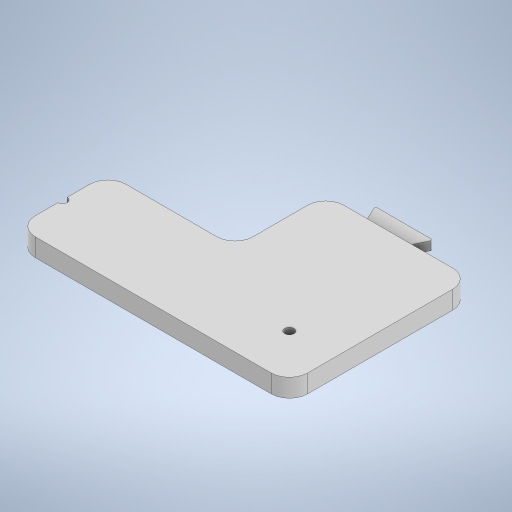
# Autodesk Inventor part: Area nh
Saved by Autodesk Inventor 2024 (Build 280153000, 153)
## iProperties
Created: 2024-03-01
Part Number: Area nh
Material: Generic
Document SubType Name: Modeling
Designer: laura
Density: 1 g/cm^3
Appearance: Default
Author: laura
Autodesk Inventor part; units mm, degrees
ref_plane "YZ Plane" through (0, 0, 0) normal (1, 0, 0) x (0, 1, 0)
ref_plane "XZ Plane" through (0, 0, 0) normal (0, 1, 0) x (-1, 0, 0)
ref_plane "XY Plane" through (0, 0, 0) normal (0, 0, 1) x (1, 0, 0)
sketch "Sketch1" plane through (0, 0, 0) normal (0, 1, 0) x (-1, 0, 0)
  line L0 (0, 0) -> (200, 0)
  line L1 (200, 0) -> (200, -150)
  line L2 (200, -150) -> (0, -150)
  line L3 (0, -150) -> (0, 0)
  dimension "d0" = 200
  dimension "d1" = 150
  constraints: 8 end point, 2 parallel, 1 horizontal, 1 perpendicular
  measures "d0" distance of L1.end L2.end
  measures "d1" distance of L0.end L1.end
extrude "Extrusion1" add sketch "Sketch1" along normal blind 10
sketch "Sketch2" plane through (0, 0, 0) normal (0, -1, 0) x (1, 0, 0)
  line L0 (-199.8, -85) -> (-186.3697, -85) construction
  line L1 (-187.7125, -90.8572) -> (-200, -85.1274)
  line L2 (-200, -85.1274) -> (-200, -64.8726)
  line L3 (-200, -64.8726) -> (-187.7125, -59.1428)
  arc A0 (-186.0054, -60.2304) -> (-187.7125, -59.1428) centre (-187.2054, -60.2304) ccw
  line L4 (-186.0054, -60.2304) -> (-186.0054, -75)
  line L5 (-186.0054, -75) -> (-186.0054, -89.7696)
  arc A1 (-187.7125, -90.8572) -> (-186.0054, -89.7696) centre (-187.2054, -89.7696) ccw
  line L6 (-200, -150) -> (-200, 0) projected
  point P0 (0, 0)
  point P1 (-186.2054, -91.3393)
  point P2 (-200, -75)
  point P3 (-200, -75)
  dimension "d4" = 15
  constraints: 12 end point, 4 point on circle, 2 centre point, 2 midpoint, 1 horizontal
  measures "d4" distance of L0.start point (-186.205, -91.339)
extrude "Extrusion2" cut sketch "Sketch2" against normal blind 5.2
sketch "Sketch3" plane through (0, 0, 0) normal (0, -1, 0) x (1, 0, 0)
  line L0 (-110, -149.8) -> (-110, -163.2303) construction
  line L1 (-100, -163.1946) -> (-114.7696, -163.1946)
  arc A0 (-115.4946, -162.0565) -> (-114.7696, -163.1946) centre (-114.7696, -162.3946) ccw
  line L2 (-115.4946, -162.0565) -> (-109.8726, -150)
  line L3 (-109.8726, -150) -> (-90.1274, -150)
  line L4 (-90.1274, -150) -> (-84.5054, -162.0565)
  arc A1 (-85.2304, -163.1946) -> (-84.5054, -162.0565) centre (-85.2304, -162.3946) ccw
  line L5 (-85.2304, -163.1946) -> (-100, -163.1946)
  line L6 (0, -150) -> (-200, -150) projected
  point P0 (0, 0)
  point P1 (-100, -150)
  point P2 (-100, -150)
  point P3 (-100, -150)
  constraints: 12 end point, 4 point on circle, 2 centre point, 2 midpoint
extrude "Extrusion3" add sketch "Sketch3" against normal blind 4.8
sketch "Sketch4" plane through (0, 10, 0) normal (0, 1, 0) x (1, 0, 0)
  line L0 (-200, 85.1274) -> (-200, 64.8726) projected
  line L1 (0, 0) -> (0, 150) projected
  line L2 (0, 75) -> (-75, 75)
  circle A0 centre (-200, 75) radius 2.6
  circle A1 centre (-75, 75) radius 2.6
  dimension "d12" = 75
  dimension "d13" = 5.2
  dimension "d14" = 5.2
  constraints: 2 centre point, 2 coincident, 2 end point, 2 midpoint, 1 horizontal
  measures "d12" distance of L2.start L2.end
  measures "d13" diameter of A0
  measures "d14" diameter of A1
extrude "Extrusion4" cut sketch "Sketch4" against normal blind 5.2
sketch "Sketch5" plane through (0, 10, 0) normal (0, 1, 0) x (1, 0, 0)
  line L0 (-200, 0) -> (0, 0) projected
  line L1 (0, 150) -> (-50, 150)
  line L2 (-50, 150) -> (-50, 0)
  line L3 (-50, 0) -> (0, 0)
  line L4 (0, 0) -> (0, 150)
  line L5 (-200, 0) -> (0, 0)
  line L6 (0, 0) -> (0, 50)
  line L7 (0, 50) -> (-200, 50)
  line L8 (-200, 50) -> (-200, 0)
  line L9 (-200, 150) -> (-130, 150)
  line L10 (-130, 150) -> (-130, 100)
  line L11 (-130, 100) -> (-200, 100)
  line L12 (-200, 100) -> (-200, 150)
  point P0 (-50, 50)
  dimension "d17" = 50
  dimension "d18" = 50
  dimension "d19" = 70
  dimension "d20" = 50
  constraints: 24 end point, 6 parallel, 3 horizontal, 3 perpendicular, 3 point on line
  measures "d17" distance of L3.end L2.end
  measures "d18" distance of L6.end L5.end
  measures "d19" distance of L10.end L11.end
  measures "d20" distance of L9.end L10.end
extrude "Extrusion5" cut sketch "Sketch5" against normal blind 15
fillet "Fillet1" radius 10 6 edges at (-50, 5, -150) (-130, 5, -150) (-200, 5, -100) (-130, 5, -100) (-200, 5, -50) (-50, 5, -50)
body "Solid1"
